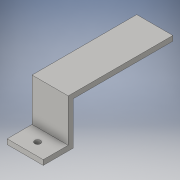
# Autodesk Inventor part: Battery Mount
Saved by Autodesk Inventor 2016 (Build 200138000, 138)
## iProperties
Created: 2017-10-13
Part Number: Battery Mount
Material: Generic
Document SubType Name: Modeling
Designer: Student
Density: 1 g/cm^3
Appearance: Default
Author: Student
Autodesk Inventor part; units mm, degrees
ref_plane "YZ Plane" through (0, 0, 0) normal (1, 0, 0) x (0, 1, 0)
ref_plane "XZ Plane" through (0, 0, 0) normal (0, 1, 0) x (-1, 0, 0)
ref_plane "XY Plane" through (0, 0, 0) normal (0, 0, 1) x (1, 0, 0)
sketch "Sketch1" plane through (0, 0, 0) normal (1, 0, 0) x (0, 1, 0)
  line L0 (0.979, 1.6933) -> (0.979, 14.3933)
  line L1 (0.979, 14.3933) -> (3.519, 14.3933)
  line L2 (3.519, 14.3933) -> (3.519, 1.6933)
  line L3 (3.519, 1.6933) -> (25.3145, 1.6933)
  line L4 (25.3145, 1.6933) -> (25.3145, -0.8467)
  line L5 (22.7745, -0.8467) -> (0.979, -0.8467)
  line L6 (0.979, -0.8467) -> (0.979, 1.6933)
  line L7 (22.7745, -0.8467) -> (22.7745, -51.6467)
  line L8 (22.7745, -51.6467) -> (25.3145, -51.6467)
  line L9 (25.3145, -51.6467) -> (25.3145, -0.8467)
  point P0 (0, 0)
  dimension "d0" = 12.7
  dimension "d1" = 12.7
  dimension "d2" = 2.54
  dimension "d3" = 2.54
  dimension "d4" = 50.8
  dimension "d5" = 2.54
  constraints: 20 end point, 4 parallel, 2 perpendicular, 1 horizontal, 1 vertical
  measures "d0" distance of L2.end L1.end
  measures "d1" distance of L0.start L0.end
  measures "d2" distance of L0.end L1.end
  measures "d3" distance of L3.end L4.end
  measures "d4" distance of L8.end L4.end
  measures "d5" distance of L7.end L8.end
extrude "Extrusion1" add sketch "Sketch1" along normal blind 18.415
sketch "Sketch2" plane through (0, 3.519, 14.3933) normal (0, 1, 0) x (1, 0, 0)
  circle A0 centre (9.2075, 6.35) radius 1.5
  line L0 (18.415, 12.7) -> (18.415, 0) projected
  line L1 (0, 0) -> (18.415, 0) projected
  point P0 (0, 14.3933)
  point P1 (18.415, 6.35)
  point P2 (9.2075, 0)
  dimension "d8" = 3
  constraints: 2 midpoint, 1 centre point, 1 horizontal alignment, 1 vertical alignment
  measures "d8" diameter of A0
extrude "Extrusion2" cut sketch "Sketch2" against normal blind 18.415
body "Solid1"
